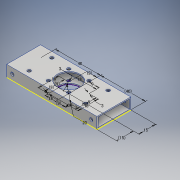
# Autodesk Inventor part: モーターパーツ１
Saved by Autodesk Inventor 2018 (Build 220112000, 112)
## iProperties
Created: 2019-04-22
Part Number: モーターパーツ１
Material: アルミニウム 6061
Document SubType Name: Modeling
Designer: Eiji Nishizawa
Density: 2.7 g/cm^3
Appearance: アルミニウム - フラット
Author: Eiji Nishizawa
Autodesk Inventor part; units mm, degrees
ref_plane "YZ Plane" through (0, 0, 0) normal (1, 0, 0) x (0, 1, 0)
ref_plane "XZ Plane" through (0, 0, 0) normal (0, 1, 0) x (-1, 0, 0)
ref_plane "XY Plane" through (0, 0, 0) normal (0, 0, 1) x (1, 0, 0)
sketch "スケッチ1" plane through (0, 0, 0) normal (1, 0, 0) x (0, 1, 0)
  line L0 (5, 5) -> (-25, 5)
  line L1 (-25, 5) -> (-25, -5)
  line L2 (-25, -5) -> (5, -5)
  line L3 (5, -5) -> (5, 5)
  line L4 (4, 4) -> (-24, 4)
  line L5 (-24, 4) -> (-24, -4)
  line L6 (-24, -4) -> (4, -4)
  line L7 (4, -4) -> (4, 4)
  point P0 (0, 0)
  dimension "d0" = 1
  dimension "d1" = 1
  dimension "d2" = 1
  dimension "d3" = 1
  dimension "d4" = 10
  dimension "d5" = 30
  dimension "d6" = 5
  dimension "d7" = 5
  constraints: 16 end point, 4 parallel, 2 horizontal, 2 perpendicular
  measures "d0" distance between parallel lines of L3 L7
  measures "d1" distance between parallel lines of L1 L5
  measures "d2" distance between parallel lines of L0 L4
  measures "d3" distance between parallel lines of L2 L6
  measures "d4" distance between parallel lines of L2 L0
  measures "d5" distance of L0.start L0.end
  measures "d6" distance from line of point (0, 0) L3
  measures "d7" distance from line of point (0, 0) L0
extrude "押し出し1" add sketch "スケッチ1" along normal blind 80
sketch "スケッチ2" plane through (0, -25, -5) normal (0, 0, -1) x (-1, 0, 0)
  circle A0 centre (-40, 15) radius 10
  line L0 (0, 30) -> (-80, 30) projected
  line L1 (0, 0) -> (-80, 0) projected
  line L2 (0, 0) -> (0, 30) projected
  line L3 (-80, 0) -> (-80, 30) projected
  circle A1 centre (-49, 24) radius 1.5
  circle A2 centre (-31, 24) radius 1.5
  circle A3 centre (-49, 6) radius 1.5
  circle A4 centre (-31, 6) radius 1.5
  point P0 (0, 25)
  dimension "d10" = 20
  dimension "d11" = 15
  dimension "d12" = 15
  dimension "d13" = 40
  dimension "d14" = 40
  dimension "d15" = 3
  dimension "d16" = 3
  dimension "d17" = 3
  dimension "d18" = 3
  dimension "d19" = 18
  dimension "d20" = 0
  dimension "d21" = 18
  dimension "d22" = 18
  dimension "d23" = 18
  dimension "d24" = 0
  dimension "d25" = 9
  dimension "d26" = 9
  dimension "d27" = 9
  dimension "d28" = 9
  dimension "d29" = 9
  dimension "d30" = 9
  dimension "d31" = 9
  constraints: 5 centre point
  measures "d10" diameter of A0
  measures "d11" distance from line of L0 A0.centre
  measures "d12" distance from line of L1 A0.centre
  measures "d13" distance from line of L2 A0.centre
  measures "d14" distance from line of A0.centre L3
  measures "d15" diameter of A1
  measures "d16" diameter of A2
  measures "d17" diameter of A3
  measures "d18" diameter of A4
  measures "d19" distance of A3.centre A1.centre
  measures "d20" vertical distance of A4.centre A3.centre
  measures "d21" distance of A2.centre A4.centre
  measures "d22" distance of A2.centre A1.centre
  measures "d23" distance of A4.centre A3.centre
  measures "d24" horizontal distance of A4.centre A2.centre
  measures "d25" horizontal distance of A0.centre A1.centre
  measures "d26" horizontal distance of A0.centre A2.centre
  measures "d27" horizontal distance of A0.centre A1.centre
  measures "d28" horizontal distance of A0.centre A3.centre
  measures "d29" horizontal distance of A0.centre A2.centre
  measures "d30" horizontal distance of A0.centre A4.centre
  measures "d31" horizontal distance of A3.centre A0.centre
extrude "押し出し2" cut sketch "スケッチ2" against normal blind 60 contours A0 | A1 | A2 | A3 | A4
sketch "スケッチ3" plane through (0, -25, -5) normal (0, -1, 0) x (1, 0, 0)
  circle A0 centre (5, 5) radius 1.5
  circle A1 centre (75, 5) radius 1.5
  line L0 (0, 10) -> (0, 0) projected
  line L1 (0, 0) -> (80, 0) projected
  line L2 (80, 10) -> (80, 0) projected
  point P0 (0, 5)
  dimension "d34" = 5
  dimension "d35" = 5
  dimension "d36" = 3
  dimension "d37" = 5
  dimension "d38" = 3
  dimension "d39" = 5
  constraints: 2 centre point
  measures "d34" distance from line of L0 A0.centre
  measures "d35" distance from line of L1 A0.centre
  measures "d36" diameter of A0
  measures "d37" distance from line of L2 A1.centre
  measures "d38" diameter of A1
  measures "d39" distance from line of L1 A1.centre
extrude "押し出し3" cut sketch "スケッチ3" against normal blind 60
sketch "スケッチ4" plane through (0, -25, -5) normal (0, 0, -1) x (-1, 0, 0)
  circle A0 centre (-15, 5) radius 1.5
  circle A1 centre (-15, 25) radius 1.5
  circle A2 centre (-65, 5) radius 1.5
  circle A3 centre (-65, 25) radius 1.5
  line L0 (0, 0) -> (0, 30) projected
  line L1 (-80, 0) -> (-80, 30) projected
  line L2 (0, 0) -> (-80, 0) projected
  line L3 (0, 30) -> (-80, 30) projected
  point P0 (0, 25)
  dimension "d42" = 3
  dimension "d43" = 3
  dimension "d44" = 15
  dimension "d45" = 15
  dimension "d46" = 15
  dimension "d47" = 15
  dimension "d48" = 3
  dimension "d49" = 3
  dimension "d50" = 5
  dimension "d51" = 5
  dimension "d52" = 5
  dimension "d53" = 5
  constraints: 4 centre point
  measures "d42" diameter of A0
  measures "d43" diameter of A1
  measures "d44" distance from line of L0 A0.centre
  measures "d45" distance from line of L0 A1.centre
  measures "d46" distance from line of L1 A2.centre
  measures "d47" distance from line of L1 A3.centre
  measures "d48" diameter of A3
  measures "d49" diameter of A2
  measures "d50" distance from line of L2 A0.centre
  measures "d51" distance from line of L2 A2.centre
  measures "d52" distance from line of L3 A1.centre
  measures "d53" distance from line of L3 A3.centre
extrude "押し出し4" cut sketch "スケッチ4" against normal blind 43 contours A0 | A1 | A2 | A3
